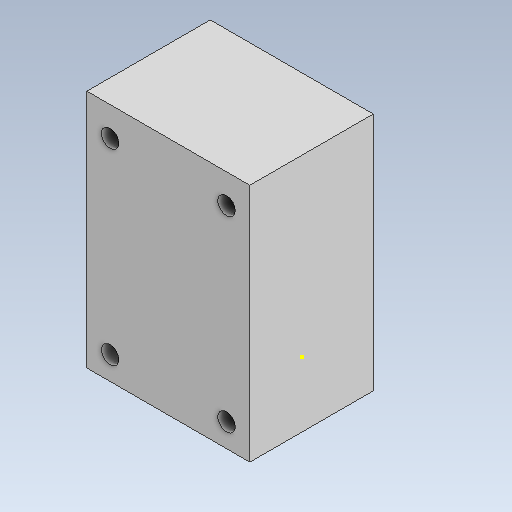
# Autodesk Inventor part: Transmission Clamp
Saved by Autodesk Inventor 2020 (Build 240168000, 168)
## iProperties
Created: 2020-03-18
Part Number: Transmission Clamp
Material: Generic
Document SubType Name: Modeling
Designer: DasNick
Density: 1 g/cm^3
Appearance: Default
Author: DasNick
Autodesk Inventor part; units mm, degrees
ref_plane "YZ Plane" through (0, 0, 0) normal (1, 0, 0) x (0, 1, 0)
ref_plane "XZ Plane" through (0, 0, 0) normal (0, 1, 0) x (-1, 0, 0)
ref_plane "XY Plane" through (0, 0, 0) normal (0, 0, 1) x (1, 0, 0)
sketch "Sketch1" plane through (0, 0, 0) normal (0, 0, 1) x (1, 0, 0)
  line L0 (-12.7, 528.7976) -> (-12.7, -380.5224)
  line L1 (12.7, 528.7976) -> (12.7, -380.5224)
  circle A0 centre (-30.0251, 19.05) radius 2.3813 projected
  circle A1 centre (-30.0251, 0) radius 2.3813 projected
  circle A2 centre (-30.0251, -19.05) radius 2.3813 projected
  line L2 (-14.1501, -31.886) -> (-58.6001, -31.886)
  line L3 (-58.6001, -31.886) -> (-58.6001, 33.5086)
  line L4 (-58.6001, 33.5086) -> (-14.1501, 33.5086)
  line L5 (-14.1501, 33.5086) -> (-14.1501, -31.886)
  line L6 (-25.1651, -297.4161) -> (-25.1651, -366.8339) projected
  point P0 (0, 0)
  dimension "d0" = 15.875
  dimension "d1" = 28.575
  constraints: 12 end point, 2 parallel, 2 vertical, 1 horizontal, 1 perpendicular, 4 other
  measures "d0" distance from line of L5 A2.centre
  measures "d1" distance from line of L3 A2.centre
extrude "Extrusion1" add sketch "Sketch1" along normal blind 33.655
sketch "Sketch2" plane through (0, 0, 33.655) normal (0, 0, 1) x (1, 0, 0)
  circle A0 centre (-30.0251, -19.05) radius 2.3813 projected
  circle A1 centre (-30.0251, 0) radius 2.3813 projected
  circle A2 centre (-30.0251, 19.05) radius 2.3813 projected
  point P0 (0, 0)
extrude "Extrusion2" add sketch "Sketch2" against normal blind 6.35
sketch "Sketch3" plane through (0, 0, 33.655) normal (0, 0, 1) x (1, 0, 0)
  circle A0 centre (-52.2501, -25.536) radius 2.3813
  line L0 (-58.6001, 33.5086) -> (-58.6001, -31.886) construction
  line L1 (-58.6001, 0) -> (-1.0342, 0) construction
  line L2 (-58.6001, -31.886) -> (-14.1501, -31.886) construction
  line L3 (-36.3751, -31.886) -> (-36.3751, 36.9987) construction
  circle A1 centre (-30.0251, -19.05) radius 2.3813 construction
  circle A2 centre (-30.0251, 0) radius 2.3813 construction
  circle A3 centre (-30.0251, 19.05) radius 2.3813 construction
  circle A4 centre (-52.2501, 25.536) radius 2.3813
  circle A5 centre (-20.5001, -25.536) radius 2.3813
  circle A6 centre (-20.5001, 25.536) radius 2.3813
  point P0 (0, 0)
  dimension "d6" = 4.7625
  dimension "d7" = 6.35
  dimension "d8" = 6.35
  constraints: 4 centre point, 4 end point, 3 symmetric about line, 1 horizontal, 1 midpoint, 1 point on line, 1 vertical, 3 other
  measures "d6" diameter of A0
  measures "d7" distance from line of L2 A0.centre
  measures "d8" distance from line of L0 A0.centre
extrude "Extrusion3" cut sketch "Sketch3" against normal blind 19.05
sketch "Sketch4" plane through (0, 0, 33.655) normal (0, 0, 1) x (1, 0, 0)
  point P0 (0, 0)
body "Solid1"
